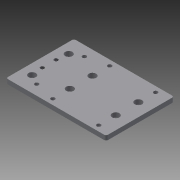
# Autodesk Inventor part: TopSupport
Saved by Autodesk Inventor 2015 SP1 (Build 190203100, 203)
## iProperties
Created: 2015-09-23
Part Number: TopSupport
Material: Generic
Document SubType Name: Modeling
Designer: I Rabey
Density: 1 g/cm^3
Appearance: Default
Author: I Rabey
Autodesk Inventor part; units mm, degrees
ref_plane "YZ Plane" through (0, 0, 0) normal (1, 0, 0) x (0, 1, 0)
ref_plane "XZ Plane" through (0, 0, 0) normal (0, 1, 0) x (-1, 0, 0)
ref_plane "XY Plane" through (0, 0, 0) normal (0, 0, 1) x (1, 0, 0)
sketch "Sketch1" plane through (0, 0, 0) normal (0, 1, 0) x (-1, 0, 0)
  line L0 (52.5, 37) -> (-52.5, 37)
  line L1 (-54.5, 35) -> (-54.5, -35)
  line L2 (-52.5, -37) -> (52.5, -37)
  line L3 (54.5, -35) -> (54.5, 35)
  line L4 (54.5, 37) -> (-54.5, -37) construction
  line L5 (-54.5, 37) -> (54.5, -37) construction
  circle A0 centre (-40.5, -31) radius 2.15
  circle A1 centre (-40.5, 31) radius 2.15
  circle A2 centre (9.5, -31) radius 2.15
  circle A3 centre (9.5, 31) radius 2.15
  circle A4 centre (32.1, 26) radius 2.15
  circle A5 centre (32.1, -26) radius 2.15
  circle A6 centre (9.6, 12.319) radius 3.95
  circle A7 centre (9.6, -12.319) radius 3.95
  circle A8 centre (-40.4, 12.319) radius 3.95
  circle A9 centre (-40.4, -12.319) radius 3.95
  circle A10 centre (43.1, 19.95) radius 3.95
  circle A11 centre (43.1, -19.95) radius 3.95
  arc A12 (54.5, 35) -> (52.5, 37) centre (52.5, 35) ccw
  arc A13 (52.5, -37) -> (54.5, -35) centre (52.5, -35) ccw
  arc A14 (-54.5, -35) -> (-52.5, -37) centre (-52.5, -35) ccw
  arc A15 (-52.5, 37) -> (-54.5, 35) centre (-52.5, 35) ccw
  circle A16 centre (44.5, -7.5) radius 2
  circle A17 centre (44.5, 7.5) radius 2
  point P0 (0, 0)
  dimension "d0" = 109
  dimension "d1" = 74
  dimension "d2" = 4.3
  dimension "d3" = 6
  dimension "d4" = 14
  dimension "d5" = 4.3
  dimension "d6" = 6
  dimension "d7" = 14
  dimension "d8" = 4.3
  dimension "d9" = 6
  dimension "d10" = 64
  dimension "d11" = 4.3
  dimension "d12" = 6
  dimension "d13" = 64
  dimension "d14" = 4.3
  dimension "d20" = 7.9
  dimension "d22" = 7.9
  dimension "d24" = 64.1
  dimension "d25" = 64.1
  dimension "d26" = 7.9
  dimension "d27" = 50
  dimension "d28" = 24.638
  dimension "d29" = 12.319
  dimension "d30" = 12.319
  dimension "d31" = 7.9
  dimension "d32" = 24.638
  dimension "d33" = 50
  dimension "d34" = 7.9
  dimension "d35" = 7.9
  dimension "d36" = 39.9
  dimension "d37" = 19.95
  dimension "d42" = 2
  dimension "d59" = 11
  dimension "d61" = 26
  dimension "d63" = 52
  dimension "d64" = 11
  dimension "d65" = 4.3
  dimension "d66" = 33.5
  dimension "d67" = 33.5
  dimension "d70" = 4
  dimension "d71" = 4
  dimension "d72" = 15
  dimension "d73" = 7.5
  dimension "d74" = 10
  dimension "d75" = 10
  constraints: 18 centre point, 12 end point, 8 point on circle, 8 point on line, 8 tangent, 3 equal radius, 2 midpoint, 2 parallel, 1 horizontal, 1 perpendicular
  measures "d0" distance of L5.end L4.end
  measures "d1" distance of L4.end L5.start
  measures "d2" diameter of A0
  measures "d3" distance from line of L2 A0.centre
  measures "d4" distance from line of L1 A0.centre
  measures "d5" diameter of A1
  measures "d6" distance from line of L0 A1.centre
  measures "d7" distance from line of L1 A1.centre
  measures "d8" diameter of A2
  measures "d9" distance from line of L2 A2.centre
  measures "d10" distance from line of L1 A2.centre
  measures "d11" diameter of A3
  measures "d12" distance from line of L0 A3.centre
  measures "d13" distance from line of L1 A3.centre
  measures "d14" diameter of A4
  measures "d20" diameter of A6
  measures "d22" diameter of A7
  measures "d24" distance from line of L1 A7.centre
  measures "d25" distance from line of L1 A6.centre
  measures "d26" diameter of A8
  measures "d27" distance of A6.centre A8.centre
  measures "d28" distance of A7.centre A6.centre
  measures "d29" vertical distance of point (0, 0) A6.centre
  measures "d30" vertical distance of point (0, 0) A8.centre
  measures "d31" diameter of A9
  measures "d32" distance of A9.centre A8.centre
  measures "d33" distance of A7.centre A9.centre
  measures "d34" diameter of A10
  measures "d35" diameter of A11
  measures "d36" distance of A11.centre A10.centre
  measures "d37" vertical distance of point (0, 0) A10.centre
  measures "d42" radius of A12
  measures "d59" horizontal distance of A4.centre A10.centre
  measures "d61" vertical distance of point (0, 0) A4.centre
  measures "d63" distance of A5.centre A4.centre
  measures "d64" horizontal distance of A5.centre A11.centre
  measures "d65" diameter of A5
  measures "d66" horizontal distance of A6.centre A10.centre
  measures "d67" horizontal distance of A7.centre A11.centre
  measures "d70" diameter of A16
  measures "d71" diameter of A17
  measures "d72" distance of A17.centre A16.centre
  measures "d73" vertical distance of point (0, 0) A17.centre
  measures "d74" distance from line of L3 A16.centre
  measures "d75" distance from line of L3 A17.centre
extrude "Extrusion5" add sketch "Sketch1" along normal blind 5
thread "Thread1" size "M4x0.7" class "6H" standard "ANSI Metric M Profile" full length
thread "Thread2" size "M4x0.7" class "6H" standard "ANSI Metric M Profile" full length
body "Solid5"
